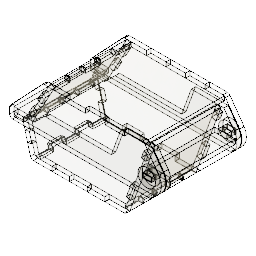
DisketteBox (Autodesk Fusion 360 design; units mm, degrees)
Autodesk Fusion 360 part; units mm, degrees
note: some values were not read from the file. Chosen so that the rebuilt part matches the saved one: which bodies a step acts on; which face or edge a step refers to. Set by a fixed rule: which sketch regions a step uses.
sketch "ShellBottomFrontBack_Sketch" plane through (0, 0, 0) normal (0, 0, 1) x (1, 0, 0)
  line L0 (0, 0) -> (60, 0)
  line L1 (60, 0) -> (60, 45)
  line L2 (60, 45) -> (0, 45)
  line L3 (0, 45) -> (0, 0)
  line L4 (60.1, 0.0219) -> (108.1, 0.0219)
  line L5 (108.1, 0.0219) -> (108.1, 45.0219)
  line L6 (108.1, 45.0219) -> (60.1, 45.0219)
  line L7 (60.1, 45.0219) -> (60.1, 0.0219)
  line L8 (-20.1, -0.1059) -> (-0.1, -0.1059)
  line L9 (-0.1, -0.1059) -> (-0.1, 44.8941)
  line L10 (-0.1, 44.8941) -> (-20.1, 44.8941)
  line L11 (-20.1, 44.8941) -> (-20.1, -0.1059)
  line L12 (30, 45) -> (30, 0) construction
  line L13 (-20.1, 22.3941) -> (108.1, 22.5219) construction
  dimension "shellBottomDepth" = 60
  dimension "shellBottomWidth" = 45
  dimension "shellBackLength" = 48
  dimension "d6" = 45
  dimension "shellFrontLength" = 20
  dimension "d8" = 45
  dimension "d9" = 0.1
  dimension "d10" = 0.1
  measures "d6" distance of L0.start
  measures "d9" distance of L3 L9
  measures "d10" distance of L1 L7
extrude "Extrude1" add sketch "ShellBottomFrontBack_Sketch" along normal blind 3 makes body 1 at (20, 30, 0) makes body 2 at (-13.4333, 29.8941, 0) makes body 3 at (92.1, 30.0219, 0)
move_body "Move1" bodies 3 to x (0.34202, 0, 0.939693) y (0, 1, 0) z (-0.939693, 0, 0.34202) at (42.9558, -1, -55.3473)
move_body "Move2" bodies 2 to x (0.258819, 0, -0.965926) y (0, 1, 0) z (0.965926, 0, 0.258819) at (-3.639, 0, 1.2576)
move_body "Move4" bodies 2 to x (1, 0, 0) y (0, 1, 0) z (0, 0, 1) at (0.7671, 0.1059, 0.8693)
move_body "Move3" bodies 3 to x (1, 0, 0) y (0, 1, 0) z (0, 0, 1) at (-0.6922, 0.9781, 0.8457)
sketch "ShellBottomToBackFinger_Sketch" plane through (60, 0, 0) normal (1, 0, 0) x (0, 1, 0)
  line L0 (0, 0) -> (45, 0)
  line L1 (45, 0) -> (45, 3)
  line L2 (45, 3) -> (0, 3)
  line L3 (0, 3) -> (0, 0)
  line L4 (36, 0) -> (36, 3)
  line L5 (27, 0) -> (27, 3)
  line L6 (18, 0) -> (18, 3)
  line L7 (9, 0) -> (9, 3)
  dimension "d29" = 9
  dimension "d32" = -9
  dimension "d33" = 0
  measures "d29" distance of L1 L4
extrude "Extrude5" add sketch "ShellBottomToBackFinger_Sketch" along normal blind 2 contours L0 L2 L6 L7 | L0 L2 L4 L5 bodies 1
extrude "Extrude6" cut sketch "ShellBottomToBackFinger_Sketch" against normal blind 1 contours L0 L2 L3 L7 | L0 L2 L5 L6 | L0 L1 L2 L4 bodies 1
sketch "ShellBottomToFrontFinger_Sketch" plane through (0, 0, 0) normal (-1, 0, 0) x (0, -1, 0)
  line L0 (-45, 0) -> (0, 0)
  line L1 (0, 0) -> (0, 3)
  line L2 (0, 3) -> (-45, 3)
  line L3 (-45, 3) -> (-45, 0)
  line L4 (-9, 0) -> (-9, 3)
  line L5 (-18, 0) -> (-18, 3)
  line L6 (-27, 0) -> (-27, 3)
  line L7 (-36, 0) -> (-36, 3)
  dimension "d38" = 9
  dimension "d41" = -9
  dimension "d42" = 0
  measures "d38" distance of L1 L4
extrude "Extrude7" add sketch "ShellBottomToFrontFinger_Sketch" along normal blind 2 contours L0 L2 L6 L7 | L0 L2 L4 L5 bodies 1
extrude "Extrude8" cut 3 faces at (0, 6, 1) (0, 24, 1) (0, 42, 1) along direction (1, 0, 0) blind 1 on bodies 1 bodies 1
sketch "ShellFrontToBottomFinger_Sketch" plane through (-0.75, 0, 2.799) normal (0.258819, 0, -0.965926) x (0, 1, 0)
  line L0 (0, -2.2235) -> (45, -2.2235)
  line L1 (45, -2.2235) -> (45, 0.7765)
  line L2 (45, 0.7765) -> (0, 0.7765)
  line L3 (0, 0.7765) -> (0, -2.2235)
  line L4 (9, -2.2235) -> (9, 0.7765)
  line L5 (18, -2.2235) -> (18, 0.7765)
  line L6 (27, -2.2235) -> (27, 0.7765)
  line L7 (36, -2.2235) -> (36, 0.7765)
  dimension "d20" = 9
  dimension "d23" = 9
  dimension "d24" = 0
  measures "d20" distance of L3 L4
extrude "Extrude3" add sketch "ShellFrontToBottomFinger_Sketch" along normal blind 2 contours L0 L2 L3 L4 | L0 L2 L5 L6 | L0 L1 L2 L7 bodies 2
extrude "Extrude4" cut 2 faces at (-0.9659, 12, 2.7412) (-1.9319, 30, 2.4824) along direction (-0.258819, 0, 0.965926) blind 1 on bodies 2 bodies 2
sketch "ShellBackToBottomFinger_Sketch" plane through (7.9828, 0, 21.9327) normal (-0.34202, 0, -0.939693) x (0, -1, 0)
  line L0 (-45, -58.3555) -> (0, -58.3555)
  line L1 (0, -58.3555) -> (0, -55.3555)
  line L2 (0, -55.3555) -> (-45, -55.3555)
  line L3 (-45, -55.3555) -> (-45, -58.3555)
  line L4 (-36, -58.3555) -> (-36, -55.3555)
  line L5 (-27, -58.3555) -> (-27, -55.3555)
  line L6 (-18, -58.3555) -> (-18, -55.3555)
  line L7 (-9, -58.3555) -> (-9, -55.3555)
  dimension "d47" = 9
  dimension "d50" = 9
  dimension "d51" = 0
  measures "d47" distance of L3 L4
extrude "Extrude9" add sketch "ShellBackToBottomFinger_Sketch" along normal blind 2 contours L0 L2 L3 L4 | L0 L2 L5 L6 | L0 L1 L2 L7 bodies 3
extrude "Extrude10" cut 2 faces at (60.9397, 33, 2.658) (60.9397, 15, 2.658) along direction (0.34202, 0, 0.939693) blind 1 on bodies 3 bodies 3
sketch "ShellSideRight_Sketch" plane through (0, 0, 0) normal (0, 1, 0) x (1, 0, 0)
  line L0 (59, 0) -> (1, 0)
  line L1 (89.646, 0) -> (-18.2643, 0) construction
  line L2 (-8.0742, -21.5421) -> (-2.3801, -0.2917)
  line L3 (-8.0742, -21.5421) -> (-2.3801, -0.2917) construction
  line L4 (-9.6191, -27.3079) -> (-0.2003, 7.8435) construction
  line L5 (-0.0264, -22.9772) -> (-8.4587, -22.9772)
  line L6 (-8.4587, -22.9772) -> (-2.302, 0)
  line L7 (-2.302, 0) -> (62.135, -0.0946)
  line L8 (92.9232, -49.1294) -> (38.6714, -49.1294) construction
  line L9 (96.5418, -52.1294) -> (51.5903, -52.1294) construction
  line L10 (80.1685, -53.2846) -> (80.1685, -24.3171) construction
  line L11 (80.1338, -32.1294) -> (99.9898, -32.1294) construction
  line L12 (79.236, -47.0792) -> (62.135, -0.0946)
  line L13 (76.417, -48.1052) -> (53.4285, -48.1052) construction
  line L14 (59, 0) -> (59, -56.8147) construction
  line L15 (59, -48.1052) -> (81.218, -48.1052)
  line L16 (-0.0264, -22.9772) -> (7.0446, -30.0483)
  line L17 (-0.0264, -22.9772) -> (9.9736, -22.9772) construction
  line L18 (7.0446, -30.0483) -> (61.9932, -30.0483) construction
  line L19 (59, -48.1052) -> (52.4278, -30.0483)
  line L20 (7.0446, -30.0483) -> (52.4278, -30.0483)
  line L21 (81.218, -48.1052) -> (88.3489, -37.8313)
  line L22 (62.135, -0.0946) -> (87.1899, -25.0433)
  arc A0 (88.3489, -37.8313) -> (87.1899, -25.0433) centre (80.1338, -32.1294) ccw
  dimension "d57" = 3
  dimension "d59" = 20
  dimension "d60" = 45
  dimension "d61" = 10
  measures "d57" distance of L8 L9
  measures "d59" distance of L9 L11
  measures "d60" angle of L16 L17
extrude "Extrude11" add sketch "ShellSideRight_Sketch" against normal blind 3 separate body makes body 4
sketch "ShellFrontToRightSideFinger_Sketch" plane through (0, 0, 0) normal (0, -1, 0) x (1, 0, 0)
  line L0 (-8.0742, 21.5421) -> (-2.3801, 0.2917)
  line L1 (-2.3801, 0.2917) -> (0.5176, 1.0681)
  line L2 (0.5176, 1.0681) -> (-5.1764, 22.3185)
  line L3 (-5.1764, 22.3185) -> (-8.0742, 21.5421)
  line L4 (-6.3487, 15.1026) -> (-3.4509, 15.879)
  line L5 (-4.6232, 8.663) -> (-1.7255, 9.4395)
  dimension "d64" = 6.6667
  dimension "d65" = 13.3333
  measures "d64" distance of L3 L4
  measures "d65" distance of L3 L5
extrude "Extrude12" add sketch "ShellFrontToRightSideFinger_Sketch" along normal blind 3 contours L0 L2 L4 L5 bodies 2
combine "Combine1" operation cut target body 4 tool bodies 2 keep tools
sketch "ShellButtomToRightSideFinger_Sketch" plane through (0, 0, 0) normal (0, -1, 0) x (1, 0, 0)
  line L0 (1, 3) -> (1, 0)
  line L1 (1, 0) -> (59, 0)
  line L2 (59, 0) -> (59, 3)
  line L3 (59, 3) -> (1, 3)
  line L4 (12, 0) -> (12, 3)
  line L5 (-2, 3) -> (1, 3)
  line L6 (0, 0) -> (0, 4.976) construction
  line L7 (24, 0) -> (24, 3)
  line L8 (36, 0) -> (36, 3)
  line L9 (48, 0) -> (48, 3)
  dimension "d68" = 12
  dimension "d71" = 12
  dimension "d72" = 0
  measures "d68" distance of L4 L6
extrude "Extrude13" add sketch "ShellButtomToRightSideFinger_Sketch" along normal blind 3 contours L1 L3 L4 L7 | L1 L3 L8 L9 bodies 1
combine "Combine2" operation cut target body 4 tool bodies 1 keep tools
sketch "ShellButtomToRightSideFinger_Sketch (1)" plane through (0, 0, 0) normal (0, -1, 0) x (1, 0, 0)
  line L0 (62.135, 0.0946) -> (79.236, 47.0792)
  line L1 (79.236, 47.0792) -> (76.417, 48.1052)
  line L2 (76.417, 48.1052) -> (59.316, 1.1206)
  line L3 (59.316, 1.1206) -> (62.135, 0.0946)
  line L4 (65.5552, 9.4915) -> (62.7362, 10.5175)
  line L5 (68.9754, 18.8884) -> (66.1564, 19.9145)
  line L6 (77.5259, 42.3807) -> (74.7069, 43.4068)
  line L7 (75.8158, 37.6823) -> (72.9968, 38.7083)
  dimension "d75" = 10
  dimension "d76" = 20
  dimension "d77" = 5
  dimension "d78" = 10
  measures "d75" distance of L3 L4
  measures "d76" distance of L3 L5
  measures "d77" distance of L1 L6
  measures "d78" distance of L1 L7
extrude "Extrude14" add sketch "ShellButtomToRightSideFinger_Sketch (1)" along normal blind 3 contours L0 L2 L4 L5 | L0 L2 L6 L7 bodies 3
combine "Combine3" operation cut target body 4 tool bodies 3 keep tools
sketch "ShellFrontToLeftSideFinger_Sketch" plane through (0, 45, 0) normal (0, 1, 0) x (-1, 0, 0)
  line L0 (2.3801, 0.2917) -> (8.0742, 21.5421)
  line L1 (8.0742, 21.5421) -> (5.1764, 22.3185)
  line L2 (5.1764, 22.3185) -> (-0.5176, 1.0681)
  line L3 (-0.5176, 1.0681) -> (2.3801, 0.2917)
  line L4 (6.3487, 15.1026) -> (3.4509, 15.879)
  line L5 (4.6232, 8.663) -> (1.7255, 9.4395)
extrude "Extrude15" add sketch "ShellFrontToLeftSideFinger_Sketch" along normal blind 3 contours L0 L2 L4 L5 bodies 2
sketch "ShellButtomToLeftSideFinger_Sketch" plane through (0, 45, 0) normal (0, 1, 0) x (-1, 0, 0)
  line L0 (-1, 0) -> (-1, 3)
  line L1 (-1, 3) -> (-59, 3)
  line L2 (-59, 3) -> (-59, 0)
  line L3 (-59, 0) -> (-1, 0)
  line L4 (-12, 0) -> (-12, 3)
  line L5 (-24, 0) -> (-24, 3)
  line L6 (-36, 0) -> (-36, 3)
  line L7 (-48, 0) -> (-48, 3)
extrude "Extrude16" add sketch "ShellButtomToLeftSideFinger_Sketch" along normal blind 3 contours L1 L3 L4 L5 | L1 L3 L6 L7 bodies 1
sketch "ShellBackToLeftSideFinger_Sketch" plane through (0, 45, 0) normal (0, 1, 0) x (-1, 0, 0)
  line L0 (-79.236, 47.0792) -> (-62.135, 0.0946)
  line L1 (-62.135, 0.0946) -> (-59.316, 1.1206)
  line L2 (-59.316, 1.1206) -> (-76.417, 48.1052)
  line L3 (-76.417, 48.1052) -> (-79.236, 47.0792)
  line L4 (-77.5259, 42.3807) -> (-74.7069, 43.4068)
  line L5 (-75.8158, 37.6823) -> (-72.9968, 38.7083)
  line L6 (-68.9754, 18.8884) -> (-66.1564, 19.9145)
  line L7 (-65.5552, 9.4915) -> (-62.7362, 10.5175)
extrude "Extrude17" add sketch "ShellBackToLeftSideFinger_Sketch" along normal blind 3 contours L0 L2 L4 L5 | L0 L2 L6 L7 bodies 3
ref_plane "WorkPlane6" through (30, 22.5, 1.5) normal (0, -1, 0) x (1, 0, 0)
mirror "Mirror2" about plane through (30, 22.5, 1.5) normal (0, -1, 0) of bodies 4 makes body 5
sketch "ShellAxis_Sketch" plane through (0, 0, 0) normal (0, 1, 0) x (-1, 0, 0)
  line L0 (-66.1564, 19.9145) -> (-62.7362, 10.5175)
  line L1 (-62.7362, 10.5175) -> (-65.5552, 9.4915)
  line L2 (-62.135, 0.0946) -> (-48, 0.0738)
  line L3 (-48, 0.0738) -> (-48, 3)
  line L4 (-48, 3) -> (-36, 3)
  line L5 (-36, 3) -> (-36, 0.0562)
  line L6 (-36, 0.0562) -> (-24, 0.0386)
  line L7 (-24, 0.0386) -> (-24, 3)
  line L8 (-24, 3) -> (-12, 3)
  line L9 (-12, 3) -> (-12, 0.021)
  line L10 (2.302, 0) -> (4.6232, 8.663)
  line L11 (4.6232, 8.663) -> (1.7255, 9.4395)
  line L12 (1.7255, 9.4395) -> (3.4509, 15.879)
  line L13 (3.4509, 15.879) -> (6.3487, 15.1026)
  line L14 (8.4587, 22.9772) -> (0.0264, 22.9772)
  line L15 (0.0264, 22.9772) -> (-7.0446, 30.0483)
  line L16 (-7.0446, 30.0483) -> (-52.4278, 30.0483)
  line L17 (-52.4278, 30.0483) -> (-59, 48.1052)
  line L18 (-59, 48.1052) -> (-81.218, 48.1052)
  line L19 (-68.9754, 18.8884) -> (-66.1564, 19.9145)
  line L20 (-65.5552, 9.4915) -> (-68.9754, 18.8884)
  line L21 (-77.5259, 42.3807) -> (-74.7069, 43.4068)
  line L22 (-74.7069, 43.4068) -> (-72.9968, 38.7083)
  line L23 (-12, 0.021) -> (2.302, 0)
  line L24 (6.3487, 15.1026) -> (8.4587, 22.9772)
  line L25 (-72.9968, 38.7083) -> (-75.8158, 37.6823)
  line L26 (-75.8158, 37.6823) -> (-77.5259, 42.3807)
  line L27 (100.311, 30.6294) -> (69.3737, 30.6294) construction
  line L28 (100.311, 33.6294) -> (68.6233, 33.6294) construction
  line L29 (100.311, 30.6294) -> (69.3737, 30.6294) construction
  line L30 (100.311, 33.6294) -> (68.6233, 33.6294) construction
  line L31 (-100.0818, 30.6294) -> (-67.2679, 30.6294) construction
  line L32 (-100.0035, 33.6294) -> (-63.1172, 33.6294) construction
  line L33 (-80.1338, 32.1294) -> (-99.9898, 32.1294) construction
  line L34 (-75.0211, 33.6294) -> (-89.1177, 33.6294)
  line L35 (-89.1177, 33.6294) -> (-89.1177, 30.6294)
  line L36 (-89.1177, 30.6294) -> (-75.0211, 30.6294)
  line L37 (-75.0211, 30.6294) -> (-75.0211, 33.6294)
  line L38 (-80.1685, 53.2846) -> (-80.1685, 24.3171)
  dimension "d171" = 1.5
  dimension "d172" = 1.5
  measures "d171" distance of L32 L33
  measures "d172" distance of L31 L33
extrude "Extrude18" add sketch "ShellAxis_Sketch" along normal blind 45 separate body contours L34 L36 L37 L38 | L34 L35 L36 L38 makes body 6
sketch "ShellAxisToRightSideFinger_Sketch" plane through (0, 0, 0) normal (0, -1, 0) x (1, 0, 0)
  line L0 (100.311, 30.6294) -> (69.3737, 30.6294) construction
  line L1 (100.311, 33.6294) -> (68.6233, 33.6294) construction
  line L2 (75.3187, 33.6294) -> (89.0558, 33.6294)
  line L3 (89.0558, 33.6294) -> (89.0558, 30.6294)
  line L4 (89.0558, 30.6294) -> (75.3187, 30.6294)
  line L5 (75.3187, 30.6294) -> (75.3187, 33.6294)
  line L6 (83.1685, 30.6294) -> (83.1685, 33.6294)
  line L7 (80.1685, 53.2846) -> (80.1685, 24.3171)
  line L8 (77.1685, 33.6294) -> (77.1685, 30.6294)
  dimension "d167" = 1.5
  dimension "d168" = 1.5
  dimension "d169" = 3
  dimension "d170" = 3
  measures "d169" distance of L6 L7
  measures "d170" distance of L7 L8
extrude "Extrude19" add sketch "ShellAxisToRightSideFinger_Sketch" along normal blind 6 contours L2 L4 L7 L8 | L2 L4 L6 L7 bodies 6
sketch "ShellAxisToLeftSideFinger_Sketch" plane through (0, 45, 0) normal (0, 1, 0) x (-1, 0, 0)
  line L0 (-75.0211, 30.6294) -> (-75.0211, 33.6294)
  line L1 (-75.0211, 33.6294) -> (-89.1177, 33.6294)
  line L2 (-89.1177, 33.6294) -> (-89.1177, 30.6294)
  line L3 (-89.1177, 30.6294) -> (-75.0211, 30.6294)
  line L4 (-83.1685, 33.6294) -> (-83.1685, 30.6294)
  line L5 (-77.1685, 33.6294) -> (-77.1685, 30.6294)
extrude "Extrude20" add sketch "ShellAxisToLeftSideFinger_Sketch" along normal blind 6 contours L1 L3 L4 L5 bodies 6
sketch "Axis_Sketch" plane through (0, -3, 0) normal (0, -1, 0) x (1, 0, 0)
  line L0 (74.7069, 43.4068) -> (77.5259, 42.3807)
  line L1 (68.9754, 18.8884) -> (65.5552, 9.4915)
  line L2 (72.9968, 38.7083) -> (74.7069, 43.4068)
  line L3 (-2.302, 0) -> (12, 0.021)
  line L4 (12, 0.021) -> (12, 3)
  line L5 (12, 3) -> (24, 3)
  line L6 (24, 3) -> (24, 0.0386)
  line L7 (24, 0.0386) -> (36, 0.0562)
  line L8 (36, 0.0562) -> (36, 3)
  line L9 (36, 3) -> (48, 3)
  line L10 (48, 3) -> (48, 0.0738)
  line L11 (48, 0.0738) -> (62.135, 0.0946)
  line L12 (65.5552, 9.4915) -> (62.7362, 10.5175)
  line L13 (62.7362, 10.5175) -> (66.1564, 19.9145)
  line L14 (66.1564, 19.9145) -> (68.9754, 18.8884)
  line L15 (81.218, 48.1052) -> (59, 48.1052)
  line L16 (59, 48.1052) -> (52.4278, 30.0483)
  line L17 (52.4278, 30.0483) -> (7.0446, 30.0483)
  line L18 (7.0446, 30.0483) -> (-0.0264, 22.9772)
  line L19 (-0.0264, 22.9772) -> (-8.4587, 22.9772)
  line L20 (-8.4587, 22.9772) -> (-6.3487, 15.1026)
  line L21 (-6.3487, 15.1026) -> (-3.4509, 15.879)
  line L22 (-3.4509, 15.879) -> (-1.7255, 9.4395)
  line L23 (-1.7255, 9.4395) -> (-4.6232, 8.663)
  line L24 (-4.6232, 8.663) -> (-2.302, 0)
  line L25 (88.3489, 37.8313) -> (81.218, 48.1052)
  line L26 (77.5259, 42.3807) -> (75.8158, 37.6823)
  line L27 (75.8158, 37.6823) -> (72.9968, 38.7083)
  line L28 (62.135, 0.0946) -> (87.1899, 25.0433)
  arc A0 (87.1899, 25.0433) -> (88.3489, 37.8313) centre (80.1338, 32.1294) ccw
  circle A1 centre (80.1338, 32.1294) radius 6
  dimension "d176" = 12
  measures "d176" diameter of A1
extrude "Extrude21" add sketch "Axis_Sketch" along normal blind 3 separate body contours A1 makes body 7
combine "Combine4" operation cut target body 7 tool bodies 6 keep tools
move_body "Move5" bodies 7 to x (1, 0, 0) y (0, 1, 0) z (0, 0, 1) at (0, -0.5, 0)
sketch "CoverSideRight_Sketch" plane through (0, -3.5, 0) normal (0, 1, 0) x (-1, 0, 0)
  line L0 (-89.2806, 52.1293) -> (19.7908, 52.1293) construction
  line L1 (0.8549, 22.9772) -> (-16.0517, 53.9289) construction
  line L2 (13.4182, 13.1688) -> (13.4182, 44.4236) construction
  line L3 (0.8549, 22.9772) -> (14.006, 22.9772) construction
  line L4 (14.006, 25.9772) -> (-18.6977, 25.9772) construction
  line L5 (14.0145, 27.9772) -> (-12.0657, 27.9772) construction
  line L6 (13.9455, 20.9772) -> (-94.938, 20.9772) construction
  line L7 (-10.8585, 54.8517) -> (2.3616, 30.6491) construction
  line L8 (13.4182, 20.9772) -> (13.4182, 27.9772)
  line L9 (13.4182, 27.9772) -> (-9.3715, 52.1293)
  line L10 (-9.3715, 52.1293) -> (-89.2806, 52.1293)
  line L11 (13.4182, 20.9772) -> (-83.1064, 20.9772)
  line L12 (0.8549, 22.9772) -> (13.4182, 22.9772)
  line L13 (13.4182, 22.9772) -> (13.4182, 25.9351)
  line L14 (13.4182, 25.9351) -> (0.8549, 25.9351)
  line L15 (0.8549, 25.9351) -> (0.8549, 22.9772)
  line L16 (-12.4647, 53.62) -> (6.9669, 18.0458) construction
  line L17 (-11.6504, 52.1293) -> (-14.2832, 50.6912)
  line L18 (-14.2832, 50.6912) -> (0.8549, 22.9772)
  line L19 (0.8549, 22.9772) -> (3.4877, 24.4153)
  line L20 (3.4877, 24.4153) -> (-11.6504, 52.1293)
  line L21 (-78.2601, 31.3581) -> (-78.2601, 53.8664) construction
  line L22 (-78.2601, 52.1293) -> (-11.6504, 52.1293)
  line L23 (-11.6504, 52.1293) -> (-11.6504, 49.1293)
  line L24 (-11.6504, 49.1293) -> (-78.2601, 49.1293)
  line L25 (-78.2601, 49.1293) -> (-78.2601, 52.1293)
  line L26 (-77.1685, 33.6294) -> (-83.1685, 33.6294)
  line L27 (-83.1685, 30.6294) -> (-77.1685, 30.6294)
  line L28 (-80.1685, 33.6294) -> (-80.1685, 30.6294) construction
  line L29 (-77.1685, 30.6294) -> (-77.1685, 33.6294)
  line L30 (-83.1685, 30.6294) -> (-83.1685, 33.6294)
  line L31 (-77.1685, 32.1294) -> (-83.1685, 32.1294) construction
  arc A0 (-88.5223, 37.5815) -> (-87.1899, 25.0433) centre (-80.1685, 32.1294) ccw
  line L32 (-83.1064, 20.9772) -> (-87.1899, 25.0433)
  line L33 (-88.5223, 37.5815) -> (-78.2601, 52.1293)
  circle A1 centre (-80.1685, 32.1294) radius 6
  dimension "d102" = 3
  dimension "d103" = 2
  dimension "d104" = 2
  dimension "d105" = 5
  dimension "d114" = 3
  dimension "d117" = 3
  dimension "d175" = 12
  measures "d102" distance of L3 L4
  measures "d103" distance of L3 L6
  measures "d104" distance of L4 L5
  measures "d105" distance of L1 L7
  measures "d114" distance of L1 L16
  measures "d175" diameter of A1
extrude "Extrude22" add sketch "CoverSideRight_Sketch" against normal blind 3 separate body contours L8 L11 L12 L18 L24 L25 A0 L32 L33 | L8 L12 L13 L14 L19 L20 | L8 L9 L10 L14 L20 | L14 L15 L18 L20 L23 L24 | L14 L15 L19 L20 | L10 L17 L18 L22 L24 L25 | L17 L18 L23 L24 | L26 L27 L29 L30 | A1 makes body 8
extrude "Extrude23" add sketch "CoverSideRight_Sketch" along normal blind 52 separate body contours L8 L12 L13 L14 L19 L20 | L14 L15 L19 L20 makes body 9
extrude "Extrude25" add sketch "CoverSideRight_Sketch" along normal blind 52 separate body contours L14 L15 L18 L20 L23 L24 | L14 L15 L19 L20 | L17 L18 L23 L24 makes body 10
extrude "Extrude26" add sketch "CoverSideRight_Sketch" along normal blind 52 separate body contours L10 L17 L18 L22 L24 L25 | L17 L18 L23 L24 makes body 11
fillet "Fillet2" radius 2 6 edges at (62.135, -1.5, 0.0946) (-2.302, -1.5, 0) (-8.4587, -1.5, 22.9772) (7.0446, -1.5, 30.0483) (59, -1.5, 48.1052) (81.218, -1.5, 48.1052) on bodies 4
sketch "CoverTopToFrontFinger_Sketch" plane through (11.6504, 0, 0) normal (-1, 0, 0) x (0, -1, 0)
  line L0 (3.5, 49.1293) -> (3.5, 52.1293)
  line L1 (3.5, 52.1293) -> (-48.5, 52.1293)
  line L2 (-48.5, 52.1293) -> (-48.5, 49.1293)
  line L3 (-48.5, 49.1293) -> (3.5, 49.1293)
  line L4 (-38.1, 49.1293) -> (-38.1, 52.1293)
  line L5 (-27.7, 49.1293) -> (-27.7, 52.1293)
  line L6 (-17.3, 49.1293) -> (-17.3, 52.1293)
  line L7 (-6.9, 49.1293) -> (-6.9, 52.1293)
  dimension "d120" = 10.4
  dimension "d123" = 10.4
  dimension "d124" = 0
  measures "d120" distance of L2 L4
extrude "Extrude27" cut sketch "CoverTopToFrontFinger_Sketch" against normal blind 3 contours L0 L1 L3 L7 | L1 L3 L5 L6 | L1 L2 L3 L4 bodies 11
sketch "CoverFrontToTopFinger_Sketch" plane through (24.6082, 0, 45.0514) normal (0.479373, 0, 0.877611) x (0, 1, 0)
  line L0 (-3.5, 14.7649) -> (-3.5, 11.7649)
  line L1 (-3.5, 11.7649) -> (48.5, 11.7649)
  line L2 (48.5, 11.7649) -> (48.5, 14.7649)
  line L3 (48.5, 14.7649) -> (-3.5, 14.7649)
  line L4 (6.9, 11.7649) -> (6.9, 14.7649)
  line L5 (17.3, 11.7649) -> (17.3, 14.7649)
  line L6 (27.7, 11.7649) -> (27.7, 14.7649)
  line L7 (38.1, 11.7649) -> (38.1, 14.7649)
  dimension "d127" = 10.4
  dimension "d130" = 10.4
  dimension "d131" = 0
  measures "d127" distance of L0 L4
extrude "Extrude28" cut sketch "CoverFrontToTopFinger_Sketch" against normal blind 3 contours L1 L3 L4 L5 | L1 L3 L6 L7 bodies 10
sketch "CoverFrontToHandleFinger_Sketch" plane through (9.4701, 0, 17.3374) normal (-0.479373, 0, -0.877611) x (0, -1, 0)
  line L0 (3.5, 11.7649) -> (3.5, 14.7649)
  line L1 (3.5, 14.7649) -> (-48.5, 14.7649)
  line L2 (-48.5, 14.7649) -> (-48.5, 11.7649)
  line L3 (-48.5, 11.7649) -> (3.5, 11.7649)
  line L4 (-38.1, 11.7649) -> (-38.1, 14.7649)
  line L5 (-27.7, 11.7649) -> (-27.7, 14.7649)
  line L6 (-17.3, 11.7649) -> (-17.3, 14.7649)
  line L7 (-6.9, 11.7649) -> (-6.9, 14.7649)
extrude "Extrude29" cut sketch "CoverFrontToHandleFinger_Sketch" against normal blind 3 contours L1 L3 L6 L7 | L1 L3 L4 L5 bodies 10
sketch "CoverHandleToFrontFinger_Sketch" plane through (-0.8549, 0, 0) normal (1, 0, 0) x (0, 1, 0)
  line L0 (-3.5, 25.9351) -> (-3.5, 22.9772)
  line L1 (-3.5, 22.9772) -> (48.5, 22.9772)
  line L2 (48.5, 22.9772) -> (48.5, 25.9351)
  line L3 (48.5, 25.9351) -> (-3.5, 25.9351)
  line L4 (6.9, 22.9772) -> (6.9, 25.9351)
  line L5 (17.3, 22.9772) -> (17.3, 25.9351)
  line L6 (27.7, 22.9772) -> (27.7, 25.9351)
  line L7 (38.1, 22.9772) -> (38.1, 25.9351)
  dimension "d136" = 10.4
  dimension "d139" = 10.4
  dimension "d140" = 0
  measures "d136" distance of L0 L4
extrude "Extrude30" cut sketch "CoverHandleToFrontFinger_Sketch" against normal blind 3 contours L0 L1 L3 L4 | L1 L3 L5 L6 | L1 L2 L3 L7 bodies 9
mirror "Mirror3" about plane through (30, 22.5, 1.5) normal (0, -1, 0) of bodies 8 7 makes body 12 at (27.1129, 48.5, 31.3612) makes body 13 at (86.1263, 50.5, 31.8303)
sketch "CoverTopToSideRightFinger_Sketch" plane through (0, -3.5, 0) normal (0, -1, 0) x (1, 0, 0)
  line L0 (14.6504, 52.1293) -> (14.6504, 49.1293)
  line L1 (14.6504, 49.1293) -> (78.2601, 49.1293)
  line L2 (78.2601, 49.1293) -> (78.2601, 52.1293)
  line L3 (78.2601, 52.1293) -> (14.6504, 52.1293)
  line L4 (64.9401, 49.1293) -> (64.9401, 52.1293)
  line L5 (51.6201, 49.1293) -> (51.6201, 52.1293)
  line L6 (38.3001, 49.1293) -> (38.3001, 52.1293)
  line L7 (24.9801, 49.1293) -> (24.9801, 52.1293)
  dimension "d144" = 13.32
  dimension "d147" = -13.32
  dimension "d148" = 0
  measures "d144" distance of L2 L4
extrude "Extrude31" add sketch "CoverTopToSideRightFinger_Sketch" along normal blind 3 contours L1 L3 L6 L7 | L1 L3 L4 L5 bodies 11
sketch "CoverTopToSideLeftFinger_Sketch" plane through (0, 48.5, 0) normal (0, 1, 0) x (-1, 0, 0)
  line L0 (-14.6504, 49.1293) -> (-14.6504, 52.1293)
  line L1 (-14.6504, 52.1293) -> (-78.2601, 52.1293)
  line L2 (-78.2601, 52.1293) -> (-78.2601, 49.1293)
  line L3 (-78.2601, 49.1293) -> (-14.6504, 49.1293)
  line L4 (-64.9401, 49.1293) -> (-64.9401, 52.1293)
  line L5 (-51.6201, 49.1293) -> (-51.6201, 52.1293)
  line L6 (-38.3001, 49.1293) -> (-38.3001, 52.1293)
  line L7 (-24.9801, 49.1293) -> (-24.9801, 52.1293)
extrude "Extrude32" add sketch "CoverTopToSideLeftFinger_Sketch" along normal blind 3 contours L1 L3 L6 L7 | L1 L3 L4 L5 bodies 11
sketch "CoverFrontToSideLeftFinger_Sketch" plane through (0, 48.5, 0) normal (0, 1, 0) x (-1, 0, 0)
  line L0 (3.4877, 24.4153) -> (-11.6504, 52.1293)
  line L1 (-11.6504, 52.1293) -> (-14.2832, 50.6912)
  line L2 (-14.2832, 50.6912) -> (0.8549, 22.9772)
  line L3 (0.8549, 22.9772) -> (3.4877, 24.4153)
  line L4 (-11.2556, 45.1484) -> (-8.6228, 46.5865)
  line L5 (-8.228, 39.6055) -> (-5.5951, 41.0437)
  line L6 (-5.2003, 34.0627) -> (-2.5675, 35.5008)
  line L7 (-2.1727, 28.5199) -> (0.4601, 29.958)
  line L8 (-11.2556, 45.1484) -> (-8.6228, 46.5865)
  line L9 (-8.6228, 46.5865) -> (-5.5951, 41.0437)
  line L10 (-5.5951, 41.0437) -> (-8.228, 39.6055)
  line L11 (-8.228, 39.6055) -> (-11.2556, 45.1484)
  line L12 (-5.2003, 34.0627) -> (-2.5675, 35.5008)
  line L13 (-2.5675, 35.5008) -> (0.4601, 29.958)
  line L14 (0.4601, 29.958) -> (-2.1727, 28.5199)
  line L15 (-2.1727, 28.5199) -> (-5.2003, 34.0627)
  dimension "d153" = 6.3158
  dimension "d154" = 6.3158
  dimension "d155" = 6.3158
  dimension "d156" = 6.3158
  measures "d153" distance of L1 L4
  measures "d154" distance of L4 L5
  measures "d155" distance of L5 L6
  measures "d156" distance of L6 L7
extrude "Extrude33" add sketch "CoverFrontToSideLeftFinger_Sketch" along normal blind 3 contours L0 L2 L6 L7 L12 L13 L14 L15 | L0 L2 L4 L5 L8 L9 L10 L11 bodies 10
sketch "CoverFrontToSideRightFinger_Sketch" plane through (0, -3.5, 0) normal (0, -1, 0) x (1, 0, 0)
  line L0 (11.6504, 52.1293) -> (-3.4877, 24.4153)
  line L1 (-3.4877, 24.4153) -> (-0.8549, 22.9772)
  line L2 (-0.8549, 22.9772) -> (14.2832, 50.6912)
  line L3 (14.2832, 50.6912) -> (11.6504, 52.1293)
  line L4 (11.2556, 45.1484) -> (8.6228, 46.5865)
  line L5 (8.6228, 46.5865) -> (5.5951, 41.0437)
  line L6 (5.5951, 41.0437) -> (8.228, 39.6055)
  line L7 (8.228, 39.6055) -> (11.2556, 45.1484)
  line L8 (5.2003, 34.0627) -> (2.5675, 35.5008)
  line L9 (2.5675, 35.5008) -> (-0.4601, 29.958)
  line L10 (-0.4601, 29.958) -> (2.1727, 28.5199)
  line L11 (2.1727, 28.5199) -> (5.2003, 34.0627)
extrude "Extrude34" add sketch "CoverFrontToSideRightFinger_Sketch" along normal blind 3 contours L0 L2 L4 L5 L6 L7 | L0 L2 L8 L9 L10 L11 bodies 10
sketch "CoverHandleToSideRightFinger_Sketch" plane through (0, -3.5, 0) normal (0, -1, 0) x (1, 0, 0)
  line L0 (-3.8549, 22.9772) -> (-3.8549, 25.9351)
  line L1 (-3.8549, 25.9351) -> (-13.4182, 25.9351)
  line L2 (-13.4182, 25.9351) -> (-13.4182, 22.9772)
  line L3 (-13.4182, 22.9772) -> (-3.8549, 22.9772)
  line L4 (-10.4182, 22.9772) -> (-10.4182, 25.9351)
  dimension "d161" = 3
  measures "d161" distance of L2 L4
extrude "Extrude35" add sketch "CoverHandleToSideRightFinger_Sketch" along normal blind 3 contours L0 L1 L3 L4 bodies 9
sketch "CoverHandleToSideLeftFinger_Sketch" plane through (0, 48.5, 0) normal (0, 1, 0) x (-1, 0, 0)
  line L0 (3.8549, 25.9351) -> (3.8549, 22.9772)
  line L1 (3.8549, 22.9772) -> (13.4182, 22.9772)
  line L2 (13.4182, 22.9772) -> (13.4182, 25.9351)
  line L3 (13.4182, 25.9351) -> (3.8549, 25.9351)
  line L4 (10.4182, 22.9772) -> (10.4182, 25.9351)
extrude "Extrude36" add sketch "CoverHandleToSideLeftFinger_Sketch" along normal blind 3 contours L0 L1 L3 L4 bodies 9
combine "Combine5" operation cut target body 12 tool bodies 11 10 9 keep tools
combine "Combine6" operation cut target body 8 tool bodies 11 10 9 keep tools
fillet "Fillet3" radius 2 5 edges at (-13.4182, -5, 27.9772) (9.3715, -5, 52.1293) (78.2601, -5, 52.1293) (-13.4182, -5, 20.9772) (83.1064, -5, 20.9772) on bodies 8 12
fillet "Fillet3" radius 2 5 edges at (78.2601, 50, 52.1293) (9.3715, 50, 52.1293) (-13.4182, 50, 27.9772) (-13.4182, 50, 20.9772) (83.1064, 50, 20.9772) on bodies 8 12
combine "Combine7" operation cut target body 4 tool bodies 6 keep tools
combine "Combine8" operation cut target body 5 tool bodies 6 keep tools
combine "Combine9" operation cut target body 8 tool bodies 7 keep tools makes body 14 at (38.5497, -3.5, 35.4662)
combine "Combine10" operation cut target body 7 tool bodies 6 keep tools
combine "Combine11" operation cut target body 12 tool bodies 13 keep tools makes body 15 at (38.5497, 48.5, 35.4662)
sketch "CoverSide_Export" plane through (0, -6.5, 0) normal (0, -1, 0) x (-1, 0, 0)
  line L0 (3.8549, 22.9772) -> (3.8549, 25.9351)
  line L1 (3.8549, 25.9351) -> (10.4182, 25.9351)
  line L2 (10.4182, 25.9351) -> (10.4182, 22.9772)
  line L3 (10.4182, 22.9772) -> (3.8549, 22.9772)
  line L4 (0.4601, 29.958) -> (-2.1727, 28.5199)
  line L5 (-2.1727, 28.5199) -> (-5.2003, 34.0627)
  line L6 (-5.2003, 34.0627) -> (-2.5675, 35.5008)
  line L7 (-2.5675, 35.5008) -> (0.4601, 29.958)
  line L8 (-5.5951, 41.0437) -> (-8.228, 39.6055)
  line L9 (-8.228, 39.6055) -> (-11.2556, 45.1484)
  line L10 (-11.2556, 45.1484) -> (-8.6228, 46.5865)
  line L11 (-8.6228, 46.5865) -> (-5.5951, 41.0437)
  line L12 (-64.9401, 49.1293) -> (-64.9401, 52.1293)
  line L13 (-64.9401, 52.1293) -> (-77.2234, 52.1293)
  line L14 (-82.2805, 20.9772) -> (11.4182, 20.9772)
  line L15 (13.4182, 22.9772) -> (13.4182, 27.1826)
  line L16 (12.8729, 28.5551) -> (-8.7794, 51.5019)
  line L17 (-10.2341, 52.1293) -> (-24.9801, 52.1293)
  line L18 (-24.9801, 52.1293) -> (-24.9801, 49.1293)
  line L19 (-24.9801, 49.1293) -> (-38.3001, 49.1293)
  line L20 (-38.3001, 49.1293) -> (-38.3001, 52.1293)
  line L21 (-38.3001, 52.1293) -> (-51.6201, 52.1293)
  line L22 (-51.6201, 52.1293) -> (-51.6201, 49.1293)
  line L23 (-51.6201, 49.1293) -> (-64.9401, 49.1293)
  line L24 (-78.8577, 51.2821) -> (-88.5223, 37.5815)
  arc A0 (-88.5223, 37.5815) -> (-87.1899, 25.0433) centre (-80.1685, 32.1294) ccw
  line L25 (-87.1899, 25.0433) -> (-83.6917, 21.56)
  arc A1 (-83.6917, 21.56) -> (-82.2805, 20.9772) centre (-82.2805, 22.9772) ccw
  arc A2 (11.4182, 20.9772) -> (13.4182, 22.9772) centre (11.4182, 22.9772) ccw
  arc A3 (13.4182, 27.1826) -> (12.8729, 28.5551) centre (11.4182, 27.1826) ccw
  arc A4 (-8.7794, 51.5019) -> (-10.2341, 52.1293) centre (-10.2341, 50.1293) ccw
  arc A5 (-77.2234, 52.1293) -> (-78.8577, 51.2821) centre (-77.2234, 50.1293) ccw
  circle A6 centre (-80.1338, 32.1294) radius 6
  line L26 (3.8549, -25.9351) -> (3.8549, -22.9772)
  line L27 (3.8549, -22.9772) -> (10.4182, -22.9772)
  line L28 (10.4182, -22.9772) -> (10.4182, -25.9351)
  line L29 (10.4182, -25.9351) -> (3.8549, -25.9351)
  line L30 (-8.6228, -46.5865) -> (-11.2556, -45.1484)
  line L31 (-11.2556, -45.1484) -> (-8.228, -39.6055)
  line L32 (-8.228, -39.6055) -> (-5.5951, -41.0437)
  line L33 (-5.5951, -41.0437) -> (-8.6228, -46.5865)
  line L34 (-2.5675, -35.5008) -> (-5.2003, -34.0627)
  line L35 (-5.2003, -34.0627) -> (-2.1727, -28.5199)
  line L36 (-2.1727, -28.5199) -> (0.4601, -29.958)
  line L37 (0.4601, -29.958) -> (-2.5675, -35.5008)
  arc A7 (-82.2805, -20.9772) -> (-83.6917, -21.56) centre (-82.2805, -22.9772) ccw
  line L38 (-83.6917, -21.56) -> (-87.1899, -25.0433)
  arc A8 (-87.1899, -25.0433) -> (-88.5223, -37.5815) centre (-80.1685, -32.1294) ccw
  line L39 (-88.5223, -37.5815) -> (-78.8577, -51.2821)
  arc A9 (-78.8577, -51.2821) -> (-77.2234, -52.1293) centre (-77.2234, -50.1293) ccw
  line L40 (-77.2234, -52.1293) -> (-64.9401, -52.1293)
  line L41 (-64.9401, -52.1293) -> (-64.9401, -49.1293)
  line L42 (-64.9401, -49.1293) -> (-51.6201, -49.1293)
  line L43 (-51.6201, -49.1293) -> (-51.6201, -52.1293)
  line L44 (-51.6201, -52.1293) -> (-38.3001, -52.1293)
  line L45 (-38.3001, -52.1293) -> (-38.3001, -49.1293)
  line L46 (-38.3001, -49.1293) -> (-24.9801, -49.1293)
  line L47 (-24.9801, -49.1293) -> (-24.9801, -52.1293)
  line L48 (-24.9801, -52.1293) -> (-10.2341, -52.1293)
  arc A10 (-10.2341, -52.1293) -> (-8.7794, -51.5019) centre (-10.2341, -50.1293) ccw
  line L49 (-8.7794, -51.5019) -> (12.8729, -28.5551)
  arc A11 (12.8729, -28.5551) -> (13.4182, -27.1826) centre (11.4182, -27.1826) ccw
  line L50 (13.4182, -27.1826) -> (13.4182, -22.9772)
  arc A12 (13.4182, -22.9772) -> (11.4182, -20.9772) centre (11.4182, -22.9772) ccw
  line L51 (11.4182, -20.9772) -> (-82.2805, -20.9772)
  circle A13 centre (-80.1338, -32.1294) radius 6
sketch "Axis_Export" plane through (0, -6.5, 0) normal (0, -1, 0) x (1, 0, 0)
  line L0 (83.1685, 33.6294) -> (83.1685, 30.6294)
  line L1 (83.1685, 30.6294) -> (77.1685, 30.6294)
  line L2 (77.1685, 30.6294) -> (77.1685, 33.6294)
  line L3 (77.1685, 33.6294) -> (83.1685, 33.6294)
  circle A0 centre (80.1338, 32.1294) radius 6
sketch "CoverTop_Export" plane through (0, 0, 52.1293) normal (0, 0, 1) x (-1, 0, 0)
  line L0 (-14.6504, -48.5) -> (-14.6504, -38.1)
  line L1 (-14.6504, -38.1) -> (-11.6504, -38.1)
  line L2 (-11.6504, -38.1) -> (-11.6504, -27.7)
  line L3 (-11.6504, -27.7) -> (-14.6504, -27.7)
  line L4 (-14.6504, -27.7) -> (-14.6504, -17.3)
  line L5 (-14.6504, -17.3) -> (-11.6504, -17.3)
  line L6 (-11.6504, -17.3) -> (-11.6504, -6.9)
  line L7 (-11.6504, -6.9) -> (-14.6504, -6.9)
  line L8 (-14.6504, -6.9) -> (-14.6504, 3.5)
  line L9 (-14.6504, 3.5) -> (-24.9801, 3.5)
  line L10 (-24.9801, 3.5) -> (-24.9801, 6.5)
  line L11 (-24.9801, 6.5) -> (-38.3001, 6.5)
  line L12 (-38.3001, 6.5) -> (-38.3001, 3.5)
  line L13 (-38.3001, 3.5) -> (-51.6201, 3.5)
  line L14 (-51.6201, 3.5) -> (-51.6201, 6.5)
  line L15 (-51.6201, 6.5) -> (-64.9401, 6.5)
  line L16 (-64.9401, 6.5) -> (-64.9401, 3.5)
  line L17 (-64.9401, 3.5) -> (-78.2601, 3.5)
  line L18 (-78.2601, 3.5) -> (-78.2601, -48.5)
  line L19 (-78.2601, -48.5) -> (-64.9401, -48.5)
  line L20 (-64.9401, -48.5) -> (-64.9401, -51.5)
  line L21 (-64.9401, -51.5) -> (-51.6201, -51.5)
  line L22 (-51.6201, -51.5) -> (-51.6201, -48.5)
  line L23 (-51.6201, -48.5) -> (-38.3001, -48.5)
  line L24 (-38.3001, -48.5) -> (-38.3001, -51.5)
  line L25 (-38.3001, -51.5) -> (-24.9801, -51.5)
  line L26 (-24.9801, -51.5) -> (-24.9801, -48.5)
  line L27 (-24.9801, -48.5) -> (-14.6504, -48.5)
sketch "CoverFront_Export" plane through (-12.9578, 0, 7.0779) normal (-0.877611, 0, 0.479373) x (0, -1, 0)
  line L0 (-27.7, 22.7552) -> (-27.7, 19.7552)
  line L1 (-27.7, 19.7552) -> (-17.3, 19.7552)
  line L2 (-17.3, 19.7552) -> (-17.3, 22.7552)
  line L3 (-17.3, 22.7552) -> (-6.9, 22.7552)
  line L4 (-6.9, 22.7552) -> (-6.9, 19.7552)
  line L5 (-6.9, 19.7552) -> (3.5, 19.7552)
  line L6 (3.5, 19.7552) -> (3.5, 26.0709)
  line L7 (3.5, 26.0709) -> (6.5, 26.0709)
  line L8 (6.5, 26.0709) -> (6.5, 32.3867)
  line L9 (6.5, 32.3867) -> (3.5, 32.3867)
  line L10 (3.5, 32.3867) -> (3.5, 38.7025)
  line L11 (3.5, 38.7025) -> (6.5, 38.7025)
  line L12 (6.5, 38.7025) -> (6.5, 45.0183)
  line L13 (6.5, 45.0183) -> (3.5, 45.0183)
  line L14 (3.5, 45.0183) -> (3.5, 51.3341)
  line L15 (3.5, 51.3341) -> (-6.9, 51.3341)
  line L16 (-6.9, 51.3341) -> (-6.9, 48.3341)
  line L17 (-6.9, 48.3341) -> (-17.3, 48.3341)
  line L18 (-17.3, 48.3341) -> (-17.3, 51.3341)
  line L19 (-17.3, 51.3341) -> (-27.7, 51.3341)
  line L20 (-27.7, 51.3341) -> (-27.7, 48.3341)
  line L21 (-27.7, 48.3341) -> (-38.1, 48.3341)
  line L22 (-38.1, 48.3341) -> (-38.1, 51.3341)
  line L23 (-38.1, 51.3341) -> (-48.5, 51.3341)
  line L24 (-48.5, 51.3341) -> (-48.5, 45.0183)
  line L25 (-48.5, 45.0183) -> (-51.5, 45.0183)
  line L26 (-51.5, 45.0183) -> (-51.5, 38.7025)
  line L27 (-51.5, 38.7025) -> (-48.5, 38.7025)
  line L28 (-48.5, 38.7025) -> (-48.5, 32.3867)
  line L29 (-48.5, 32.3867) -> (-51.5, 32.3867)
  line L30 (-51.5, 32.3867) -> (-51.5, 26.0709)
  line L31 (-51.5, 26.0709) -> (-48.5, 26.0709)
  line L32 (-48.5, 26.0709) -> (-48.5, 19.7552)
  line L33 (-48.5, 19.7552) -> (-38.1, 19.7552)
  line L34 (-38.1, 19.7552) -> (-38.1, 22.7552)
  line L35 (-38.1, 22.7552) -> (-27.7, 22.7552)
sketch "CoverHandle_Export" plane through (0, 0, 25.9351) normal (0, 0, 1) x (-1, 0, 0)
  line L0 (3.8549, -6.9) -> (0.8549, -6.9)
  line L1 (0.8549, -6.9) -> (0.8549, -17.3)
  line L2 (0.8549, -17.3) -> (3.8549, -17.3)
  line L3 (3.8549, -17.3) -> (3.8549, -27.7)
  line L4 (3.8549, -27.7) -> (0.8549, -27.7)
  line L5 (0.8549, -27.7) -> (0.8549, -38.1)
  line L6 (0.8549, -38.1) -> (3.8549, -38.1)
  line L7 (3.8549, -38.1) -> (3.8549, -51.5)
  line L8 (3.8549, -51.5) -> (10.4182, -51.5)
  line L9 (10.4182, -51.5) -> (10.4182, -48.5)
  line L10 (10.4182, -48.5) -> (13.4182, -48.5)
  line L11 (13.4182, -48.5) -> (13.4182, 3.5)
  line L12 (13.4182, 3.5) -> (10.4182, 3.5)
  line L13 (10.4182, 3.5) -> (10.4182, 6.5)
  line L14 (10.4182, 6.5) -> (3.8549, 6.5)
  line L15 (3.8549, 6.5) -> (3.8549, -6.9)
sketch "ShellAxis_Export" plane through (0, 0, 33.6294) normal (0, 0, 1) x (-1, 0, 0)
  line L0 (-75.0211, 0) -> (-77.1685, 0)
  line L1 (-77.1685, 0) -> (-77.1685, 6)
  line L2 (-77.1685, 6) -> (-83.1685, 6)
  line L3 (-83.1685, 6) -> (-83.1685, 0)
  line L4 (-83.1685, 0) -> (-89.1177, 0)
  line L5 (-89.1177, 0) -> (-89.1177, -45)
  line L6 (-89.1177, -45) -> (-83.1685, -45)
  line L7 (-83.1685, -45) -> (-83.1685, -51)
  line L8 (-83.1685, -51) -> (-77.1685, -51)
  line L9 (-77.1685, -51) -> (-77.1685, -45)
  line L10 (-77.1685, -45) -> (-75.0211, -45)
  line L11 (-75.0211, -45) -> (-75.0211, 0)
sketch "ShellBack_Export" plane through (52.0172, 0, -18.9327) normal (-0.939693, 0, 0.34202) x (0, -1, 0)
  line L0 (-27, 24.3403) -> (-27, 21.3403)
  line L1 (-27, 21.3403) -> (-18, 21.3403)
  line L2 (-18, 21.3403) -> (-18, 24.3403)
  line L3 (-18, 24.3403) -> (-9, 24.3403)
  line L4 (-9, 24.3403) -> (-9, 21.3403)
  line L5 (-9, 21.3403) -> (0, 21.3403)
  line L6 (0, 21.3403) -> (0, 31.3403)
  line L7 (0, 31.3403) -> (3, 31.3403)
  line L8 (3, 31.3403) -> (3, 41.3403)
  line L9 (3, 41.3403) -> (0, 41.3403)
  line L10 (0, 41.3403) -> (0, 61.3403)
  line L11 (0, 61.3403) -> (3, 61.3403)
  line L12 (3, 61.3403) -> (3, 66.3403)
  line L13 (3, 66.3403) -> (0, 66.3403)
  line L14 (0, 66.3403) -> (0, 71.3403)
  line L15 (0, 71.3403) -> (-45, 71.3403)
  line L16 (-45, 71.3403) -> (-45, 66.3403)
  line L17 (-45, 66.3403) -> (-48, 66.3403)
  line L18 (-48, 66.3403) -> (-48, 61.3403)
  line L19 (-48, 61.3403) -> (-45, 61.3403)
  line L20 (-45, 61.3403) -> (-45, 41.3403)
  line L21 (-45, 41.3403) -> (-48, 41.3403)
  line L22 (-48, 41.3403) -> (-48, 31.3403)
  line L23 (-48, 31.3403) -> (-45, 31.3403)
  line L24 (-45, 31.3403) -> (-45, 21.3403)
  line L25 (-45, 21.3403) -> (-36, 21.3403)
  line L26 (-36, 21.3403) -> (-36, 24.3403)
  line L27 (-36, 24.3403) -> (-27, 24.3403)
sketch "ShellFront_Export" plane through (0.75, 0, 0.201) normal (0.965926, 0, 0.258819) x (0, 1, 0)
  line L0 (18, 3.8978) -> (18, 0.8978)
  line L1 (18, 0.8978) -> (27, 0.8978)
  line L2 (27, 0.8978) -> (27, 3.8978)
  line L3 (27, 3.8978) -> (36, 3.8978)
  line L4 (36, 3.8978) -> (36, 0.8978)
  line L5 (36, 0.8978) -> (45, 0.8978)
  line L6 (45, 0.8978) -> (45, 9.5644)
  line L7 (45, 9.5644) -> (48, 9.5644)
  line L8 (48, 9.5644) -> (48, 16.2311)
  line L9 (48, 16.2311) -> (45, 16.2311)
  line L10 (45, 16.2311) -> (45, 22.8978)
  line L11 (45, 22.8978) -> (0, 22.8978)
  line L12 (0, 22.8978) -> (0, 16.2311)
  line L13 (0, 16.2311) -> (-3, 16.2311)
  line L14 (-3, 16.2311) -> (-3, 9.5644)
  line L15 (-3, 9.5644) -> (0, 9.5644)
  line L16 (0, 9.5644) -> (0, 0.8978)
  line L17 (0, 0.8978) -> (9, 0.8978)
  line L18 (9, 0.8978) -> (9, 3.8978)
  line L19 (9, 3.8978) -> (18, 3.8978)
sketch "ShellBottom_Export" plane through (0, 0, 3) normal (0, 0, 1) x (-1, 0, 0)
  line L0 (-1, -18) -> (2, -18)
  line L1 (2, -18) -> (2, -9)
  line L2 (2, -9) -> (-1, -9)
  line L3 (-1, -9) -> (-1, 0)
  line L4 (-1, 0) -> (-12, 0)
  line L5 (-12, 0) -> (-12, 3)
  line L6 (-12, 3) -> (-24, 3)
  line L7 (-24, 3) -> (-24, 0)
  line L8 (-24, 0) -> (-36, 0)
  line L9 (-36, 0) -> (-36, 3)
  line L10 (-36, 3) -> (-48, 3)
  line L11 (-48, 3) -> (-48, 0)
  line L12 (-48, 0) -> (-59, 0)
  line L13 (-59, 0) -> (-59, -9)
  line L14 (-59, -9) -> (-62, -9)
  line L15 (-62, -9) -> (-62, -18)
  line L16 (-62, -18) -> (-59, -18)
  line L17 (-59, -18) -> (-59, -27)
  line L18 (-59, -27) -> (-62, -27)
  line L19 (-62, -27) -> (-62, -36)
  line L20 (-62, -36) -> (-59, -36)
  line L21 (-59, -36) -> (-59, -45)
  line L22 (-59, -45) -> (-48, -45)
  line L23 (-48, -45) -> (-48, -48)
  line L24 (-48, -48) -> (-36, -48)
  line L25 (-36, -48) -> (-36, -45)
  line L26 (-36, -45) -> (-24, -45)
  line L27 (-24, -45) -> (-24, -48)
  line L28 (-24, -48) -> (-12, -48)
  line L29 (-12, -48) -> (-12, -45)
  line L30 (-12, -45) -> (-1, -45)
  line L31 (-1, -45) -> (-1, -36)
  line L32 (-1, -36) -> (2, -36)
  line L33 (2, -36) -> (2, -27)
  line L34 (2, -27) -> (-1, -27)
  line L35 (-1, -27) -> (-1, -18)
sketch "ShellSide_Export" plane through (0, 0, 0) normal (0, 1, 0) x (-1, 0, 0)
  line L0 (2.6998, 1.4846) -> (4.6232, 8.663)
  line L1 (4.6232, 8.663) -> (1.7255, 9.4395)
  line L2 (1.7255, 9.4395) -> (3.4509, 15.879)
  line L3 (3.4509, 15.879) -> (6.3487, 15.1026)
  line L4 (5.8522, 22.9772) -> (0.0264, 22.9772)
  line L5 (0.0264, 22.9772) -> (-6.4589, 29.4625)
  line L6 (-7.8731, 30.0483) -> (-52.4278, 30.0483)
  line L7 (-52.4278, 30.0483) -> (-58.521, 46.7893)
  line L8 (-60.4004, 48.1052) -> (-80.1716, 48.1052)
  line L9 (-68.9754, 18.8884) -> (-66.1564, 19.9145)
  line L10 (-66.1564, 19.9145) -> (-62.7362, 10.5175)
  line L11 (-62.7362, 10.5175) -> (-65.5552, 9.4915)
  line L12 (-61.3108, 0.0933) -> (-48, 0.0738)
  line L13 (-48, 0.0738) -> (-48, 3)
  line L14 (-48, 3) -> (-36, 3)
  line L15 (-36, 3) -> (-36, 0.0562)
  line L16 (-36, 0.0562) -> (-24, 0.0386)
  line L17 (-24, 0.0386) -> (-24, 3)
  line L18 (-24, 3) -> (-12, 3)
  line L19 (-12, 3) -> (-12, 0.021)
  line L20 (-65.5552, 9.4915) -> (-68.9754, 18.8884)
  line L21 (-77.5259, 42.3807) -> (-74.7069, 43.4068)
  line L22 (-74.7069, 43.4068) -> (-72.9968, 38.7083)
  line L23 (-81.8146, 47.2456) -> (-88.3489, 37.8313)
  line L24 (-77.1685, 33.6294) -> (-77.1685, 30.6294)
  line L25 (-77.1685, 30.6294) -> (-83.1685, 30.6294)
  line L26 (-83.1685, 30.6294) -> (-83.1685, 33.6294)
  line L27 (-83.1685, 33.6294) -> (-77.1685, 33.6294)
  arc A0 (-88.3489, 37.8313) -> (-87.1899, 25.0433) centre (-80.1338, 32.1294) ccw
  line L28 (-87.1899, 25.0433) -> (-62.7191, 0.6761)
  line L29 (-72.9968, 38.7083) -> (-75.8158, 37.6823)
  arc A1 (-80.1716, 48.1052) -> (-81.8146, 47.2456) centre (-80.1716, 46.1052) ccw
  arc A2 (-62.7191, 0.6761) -> (-61.3108, 0.0933) centre (-61.3079, 2.0933) ccw
  line L30 (-12, 0.021) -> (0.765, 0.0023)
  arc A3 (0.765, 0.0023) -> (2.6998, 1.4846) centre (0.7679, 2.0023) ccw
  line L31 (6.3487, 15.1026) -> (7.7841, 20.4596)
  arc A4 (7.7841, 20.4596) -> (5.8522, 22.9772) centre (5.8522, 20.9772) ccw
  arc A5 (-6.4589, 29.4625) -> (-7.8731, 30.0483) centre (-7.8731, 28.0483) ccw
  arc A6 (-58.521, 46.7893) -> (-60.4004, 48.1052) centre (-60.4004, 46.1052) ccw
  line L32 (-75.8158, 37.6823) -> (-77.5259, 42.3807)
hidden bodies 12
equation "thickness = 3 mm"
equation "d6 = shellBottomWidth"
equation "d8 = shellBottomWidth"
equation "d20 = shellBottomWidth / 5"
equation "d23 = shellBottomWidth / 5"
equation "d25 = thickness / 3 * 2"
equation "d27 = -thickness / 3"
equation "d29 = shellBottomWidth / 5"
equation "d32 = -shellBottomWidth / 5"
equation "d34 = thickness / 3 * 2"
equation "d36 = -thickness / 3"
equation "d38 = shellBottomWidth / 5"
equation "d41 = -shellBottomWidth / 5"
equation "d43 = thickness / 3 * 2"
equation "d45 = -thickness / 3"
equation "d47 = shellBottomWidth / 5"
equation "d50 = shellBottomWidth / 5"
equation "d52 = thickness / 3 * 2"
equation "d54 = -thickness / 3"
equation "d57 = thickness"
equation "d62 = -thickness"
equation "d64 = shellFrontLength / 3"
equation "d65 = shellFrontLength / 3 * 2"
equation "d66 = thickness"
equation "d68 = shellBottomDepth / 5"
equation "d71 = shellBottomDepth / 5"
equation "d73 = thickness"
equation "d79 = thickness"
equation "d81 = thickness"
equation "d83 = thickness"
equation "d85 = thickness"
equation "d90 = shellBottomWidth"
equation "d94 = thickness * 2"
equation "d96 = thickness * 2"
equation "d100 = thickness"
equation "d102 = thickness"
equation "d105 = thickness + 2 mm"
equation "d106 = -thickness"
equation "d109 = shellBottomWidth + ( 2 * thickness ) + 1 mm"
equation "d114 = thickness"
equation "d115 = shellBottomWidth + ( 2 * thickness ) + 1 mm"
equation "d117 = thickness"
equation "d118 = shellBottomWidth + ( 2 * thickness ) + 1 mm"
equation "d120 = ( shellBottomWidth + ( 2 * thickness ) + 1 mm ) / 5"
equation "d123 = ( shellBottomWidth + ( 2 * thickness ) + 1 mm ) / 5"
equation "d125 = -thickness"
equation "d127 = ( shellBottomWidth + ( 2 * thickness ) + 1 mm ) / 5"
equation "d130 = ( shellBottomWidth + ( 2 * thickness ) + 1 mm ) / 5"
equation "d132 = -thickness"
equation "d134 = -thickness"
equation "d136 = ( shellBottomWidth + ( 2 * thickness ) + 1 mm ) / 5"
equation "d139 = ( shellBottomWidth + ( 2 * thickness ) + 1 mm ) / 5"
equation "d141 = -thickness"
equation "d149 = thickness"
equation "d151 = thickness"
equation "d157 = thickness"
equation "d159 = thickness"
equation "d162 = thickness"
equation "d164 = thickness"
named bodies: "ShellBottom_Body", "ShellFront_Body", "ShellBack_Body", "ShellRightSide_Body", "ShellLeftSide_Body (Mirror)", "ShellAxis_Body", "Axis_Body", "CoverRightSide_Body", "CoverHandle_Body", "CoverFront_Body", "CoverTop_Body", "CoverLeftSide_Body (Mirror)", "Axis_Body (Mirror)", "CoverRightSide_Body (1)", "CoverLeftSide_Body (Mirror) (1)"
